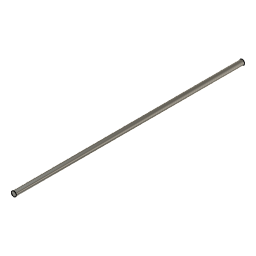
Vodící tyč - krátká v2 (Autodesk Fusion 360 design; units mm, degrees)
Autodesk Fusion 360 part; units mm, degrees
sketch "Sketch1" plane through (0, 0, 0) normal (0, 1, 0) x (1, 0, 0)
  circle A0 centre (0, 0) radius 3
  dimension "d1" = 6
  constraint coincident A0.centre origin
  measures "d1" diameter of A0
extrude "Extrude1" add sketch "Sketch1" along normal blind 336
extrude "Extrude2" cut 1 faces at (-1.1591, 0, -0.5829) along direction (0, 1, 0) blind 50
extrude "Extrude3" cut 1 faces at (-1.1591, 50, -0.5829) along direction (0, 1, 0) blind 6
